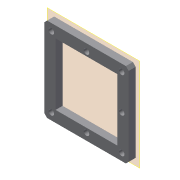
# Autodesk Inventor part: cellSTORM_v5_cellphonespacer
Saved by Autodesk Inventor 2019.4 (Build 234330000, 330)
## iProperties
Created: 2020-06-07
Part Number: cellSTORM_v5_cellphonespacer
Material: Generic
Document SubType Name: Modeling
Designer: diederichbenedict
Density: 1 g/cm^3
Appearance: Default
Author: diederichbenedict
Autodesk Inventor part; units mm, degrees
ref_plane "YZ Plane" through (0, 0, 0) normal (1, 0, 0) x (0, 1, 0)
ref_plane "XZ Plane" through (0, 0, 0) normal (0, 1, 0) x (-1, 0, 0)
ref_plane "XY Plane" through (0, 0, 0) normal (0, 0, 1) x (1, 0, 0)
ref_plane "Work Plane1" through (0, 0, -5) normal (0, 0, 1) x (1, 0, 0)
sketch "Sketch1" plane through (0, 0, -5) normal (0, 0, 1) x (1, 0, 0)
  line L0 (-45, 22) -> (22, 22) projected
  line L1 (22, 22) -> (22, -22) projected
  line L2 (22, -22) -> (-45, -22) projected
  line L3 (-45, -28) -> (-45, -22) projected
  line L4 (-30, -28) -> (-45, -28) projected
  line L5 (-30, -28) -> (-28, -30) projected
  line L6 (-28, -30) -> (28, -30) projected
  line L7 (28, -30) -> (30, -28) projected
  line L8 (30, -28) -> (30, 28) projected
  line L9 (30, 28) -> (28, 30) projected
  line L10 (28, 30) -> (-28, 30) projected
  line L11 (-28, 30) -> (-30, 28) projected
  line L12 (-30, 28) -> (-45, 28) projected
  line L13 (-45, 22) -> (-45, 28) projected
  circle A0 centre (25, 25) radius 1.95 projected
  circle A1 centre (25, 0) radius 1.95 projected
  circle A2 centre (0, 25) radius 1.95 projected
  circle A3 centre (-25, -25) radius 1.95 projected
  circle A4 centre (25, -25) radius 1.95 projected
  circle A5 centre (-25, 25) radius 1.95 projected
  circle A6 centre (0, -25) radius 1.95 projected
  line L14 (-30, 28) -> (-30, -28)
  line L15 (22, 22) -> (-22, 22)
  line L16 (-22, 22) -> (-22, -22)
  line L17 (-22, -22) -> (22, -22)
  line L18 (22, -22) -> (22, 22)
  point P0 (0, 0)
  dimension "d0" = 44
  dimension "d1" = 44
  constraints: 10 end point, 2 parallel, 1 horizontal, 1 perpendicular, 1 vertical
  measures "d0" distance of L17.end L16.end
  measures "d1" distance of L16.end L15.end
extrude "Extrusion1" add sketch "Sketch1" along normal blind 5 contours L0 L14 L11 L10 L9 L8 L7 L6 L5 L2 L1 | L16 L2 L14 L0
body "Solid1"
